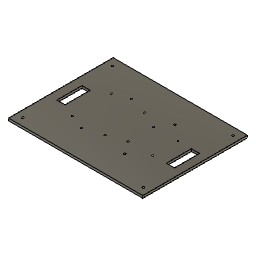
Board Tester v1 (Autodesk Fusion 360 design; units mm, degrees)
Autodesk Fusion 360 part; units mm, degrees
sketch "Sketch1" plane through (0, 0, 0) normal (0, 0, 1) x (1, 0, 0)
  circle A0 centre (-13.6792, 145.0658) radius 1.5
  circle A1 centre (165.3208, 145.0658) radius 1.5
  circle A2 centre (-13.6792, 12.1658) radius 1.5
  circle A3 centre (165.3208, 12.1658) radius 1.5
  circle A4 centre (43.3208, 42.5182) radius 1.5
  circle A5 centre (108.3208, 41.4658) radius 1.5
  circle A6 centre (43.3208, 116.7382) radius 1.5
  circle A7 centre (108.3208, 115.7658) radius 1.5
  line L0 (-23.5792, 156.1658) -> (175.3708, 156.1658)
  line L1 (175.3708, 156.1658) -> (175.3708, 1.0658)
  line L2 (175.3708, 1.0658) -> (-23.5792, 1.0658)
  line L3 (-23.5792, 1.0658) -> (-23.5792, 156.1658)
  circle A8 centre (21.2, 108.6782) radius 1.25
  circle A9 centre (70, 108.6782) radius 1.25
  circle A10 centre (21.2, 50.5782) radius 1.25
  circle A11 centre (70, 50.5782) radius 1.25
  circle A12 centre (95, 97.3658) radius 1.25
  circle A13 centre (131.3, 97.3658) radius 1.25
  circle A14 centre (95, 59.8658) radius 1.25
  circle A15 centre (131.3, 59.8658) radius 1.25
  line L4 (-10.8, 97.1908) -> (1.2, 97.1908)
  line L5 (1.2, 97.1908) -> (1.2, 60.0408)
  line L6 (1.2, 60.0408) -> (-10.8, 60.0408)
  line L7 (-10.8, 60.0408) -> (-10.8, 97.1908)
  line L8 (151.3, 97.1908) -> (163.3, 97.1908)
  line L9 (151.3, 60.0408) -> (151.3, 97.1908)
  line L10 (163.3, 60.0408) -> (151.3, 60.0408)
  line L11 (163.3, 97.1908) -> (163.3, 60.0408)
  dimension "d1" = 3
  dimension "d2" = 3
  dimension "d3" = 3
  dimension "d4" = 3
  dimension "d14" = 3
  dimension "d15" = 3
  dimension "d16" = 3
  dimension "d17" = 3
  dimension "d21" = 74.3
  dimension "d33" = 67.05
  dimension "d34" = 67.05
  dimension "d36" = 65
  dimension "d37" = 66.9
  dimension "d38" = 65
  dimension "d39" = 11.1
  dimension "d40" = 9.9
  dimension "d41" = 11.1
  dimension "d42" = 10.05
  dimension "d43" = 10.05
  dimension "d44" = 11.1
  dimension "d45" = 11.1
  dimension "d46" = 9.9
  dimension "d47" = 40.4
  dimension "d48" = 40.4
  dimension "d49" = 2.5
  dimension "d50" = 2.5
  dimension "d51" = 2.5
  dimension "d52" = 2.5
  dimension "d53" = 58.1
  dimension "d54" = 58.1
  dimension "d55" = 48.8
  dimension "d56" = 48.8
  dimension "d65" = 2.5
  dimension "d66" = 2.5
  dimension "d67" = 2.5
  dimension "d68" = 2.5
  dimension "d71" = 36.3
  dimension "d72" = 36.3
  dimension "d73" = 37.5
  dimension "d74" = 37.5
  dimension "d79" = 18.4
  dimension "d80" = 37.15
  dimension "d81" = 12
  dimension "d82" = 37.15
  dimension "d83" = 12
  dimension "d84" = 8.06
  dimension "d85" = 8.06
  dimension "d86" = 18.4
  dimension "d88" = 25
  dimension "d91" = 20
  dimension "d92" = 47.875
  dimension "d93" = 20
  dimension "d94" = 47.875
  constraint horizontal L0
  constraint vertical L1
  constraint horizontal L2
  constraint vertical L3
  constraint horizontal L4
  constraint vertical L5
  constraint horizontal L6
  constraint vertical L7
  constraint horizontal L8
  constraint vertical L11
  constraint horizontal L10
  constraint vertical L9
  measures "d1" diameter of A0
  measures "d2" diameter of A1
  measures "d3" diameter of A2
  measures "d4" diameter of A3
  measures "d14" diameter of A4
  measures "d15" diameter of A5
  measures "d16" diameter of A6
  measures "d17" diameter of A7
  measures "d21" vertical distance of A5.centre A7.centre
  measures "d33" distance of A7.centre L1
  measures "d34" distance of A5.centre L1
  measures "d36" horizontal distance of A4.centre A5.centre
  measures "d37" distance of A6.centre L3
  measures "d38" horizontal distance of A6.centre A7.centre
  measures "d39" distance of A0.centre L0
  measures "d40" distance of A0.centre L3
  measures "d41" distance of A1.centre L0
  measures "d42" distance of A1.centre L1
  measures "d43" distance of A3.centre L1
  measures "d44" distance of A3.centre L2
  measures "d45" distance of A2.centre L2
  measures "d46" distance of A2.centre L3
  measures "d47" distance of A7.centre L0
  measures "d48" distance of A5.centre L2
  measures "d49" diameter of A8
  measures "d50" diameter of A9
  measures "d51" diameter of A10
  measures "d52" diameter of A11
  measures "d53" distance of A8.centre A10.centre
  measures "d54" distance of A9.centre A11.centre
  measures "d55" distance of A8.centre A9.centre
  measures "d56" distance of A10.centre A11.centre
  measures "d65" diameter of A12
  measures "d66" diameter of A13
  measures "d67" diameter of A14
  measures "d68" diameter of A15
  measures "d71" distance of A12.centre A13.centre
  measures "d72" distance of A14.centre A15.centre
  measures "d73" distance of A12.centre A14.centre
  measures "d74" distance of A13.centre A15.centre
  measures "d79" vertical distance of A7.centre A12.centre
  measures "d80" distance of L4.start L6.end
  measures "d81" distance of L5.end L6.end
  measures "d82" distance of L8.start L9.start
  measures "d83" distance of L10.start L9.start
  measures "d84" vertical distance of A6.centre A9.centre
  measures "d85" vertical distance of A4.centre A11.centre
  measures "d86" vertical distance of A5.centre A14.centre
  measures "d88" horizontal distance of A11.centre A14.centre
  measures "d91" distance of A13.centre L9
  measures "d92" distance of A1.centre L8
  measures "d93" distance of A8.centre L5
  measures "d94" distance of A0.centre L4
extrude "Extrude1" add sketch "Sketch1" along normal blind 3.5
